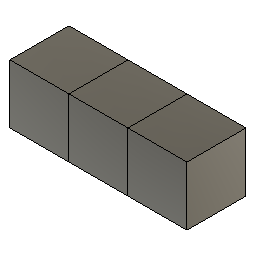
BooleanIntersectOverlap (Autodesk Fusion 360 design; units mm, degrees)
Autodesk Fusion 360 part; units mm, degrees
sketch "Sketch1" plane through (0, 0, 0) normal (0, 0, 1) x (1, 0, 0)
  line L0 (0, 0) -> (-20, 0)
  line L1 (-20, 0) -> (-20, 10)
  line L2 (-20, 10) -> (0, 10)
  line L3 (0, 10) -> (0, 0)
  constraint horizontal L0
  constraint vertical L1
  constraint horizontal L2
  constraint vertical L3
  constraint coincident L0.start L3.end
extrude "Extrude1" add sketch "Sketch1" along normal blind 10 makes body 1
sketch "Sketch1 (2)" plane through (0, 0, 0) normal (0, 0, 1) x (1, 0, 0) in component "Tool"
  line L0 (-10, 10) -> (10, 10)
  line L1 (10, 10) -> (10, 0)
  line L2 (10, 0) -> (-10, 0)
  line L3 (-10, 0) -> (-10, 10)
  constraint horizontal L0
  constraint vertical L1
  constraint horizontal L2
  constraint vertical L3
extrude "Extrude1'" add sketch "Sketch1 (2)" along normal blind 10 separate body makes body 2 in component "Tool"
component "Tool" placed x (1, 0, 0) y (0, 1, 0) z (0, 0, 1) at (0, 0, 0)
